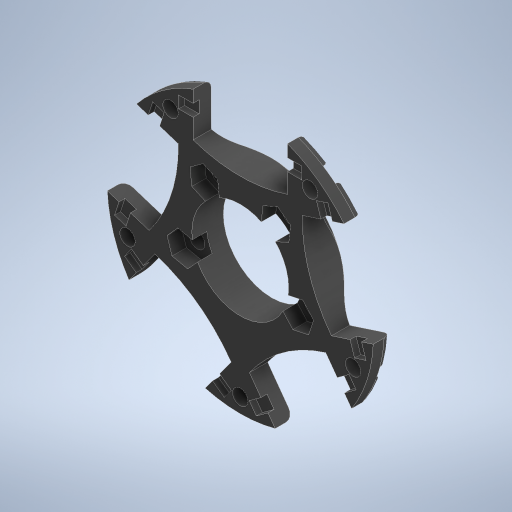
# Autodesk Inventor part: wheel_body_back_inside
Saved by Autodesk Inventor 2024.1 (Build 281209000, 209)
## iProperties
Created: 2024-11-26
Part Number: wheel_body_back_inside
Material: 一般
Document SubType Name: Modeling
Designer: hibik
Density: 1 g/cm^3
Appearance: 既定
Author: hibik
Autodesk Inventor part; units mm, degrees
ref_plane "YZ Plane" through (0, 0, 0) normal (1, 0, 0) x (0, 1, 0)
ref_plane "XZ Plane" through (0, 0, 0) normal (0, 1, 0) x (-1, 0, 0)
ref_plane "XY Plane" through (0, 0, 0) normal (0, 0, 1) x (1, 0, 0)
sketch "スケッチ1" plane through (0, 0, 0) normal (0, 0, 1) x (1, 0, 0)
  arc A0 (-9.75, 17.688144) -> (9.75, 17.688144) centre (0, 45) ccw
  arc A1 (-9.75, 16.62858) -> (9.75, 16.62858) centre (0, 45) ccw
  line L0 (-9.75, 42) -> (9.75, 42)
  line L1 (9.75, 42) -> (9.75, 15)
  line L2 (9.75, 15) -> (-9.75, 15)
  line L3 (-9.75, 15) -> (-9.75, 42)
  line L4 (-9.75, 29) -> (9.75, 29)
  circle A2 centre (0, 0) radius 10
  circle A3 centre (0, 0) radius 15 construction
  circle A4 centre (0, 0) radius 29
  line L5 (-17.278763, -4.637546) -> (-42.957289, 3.705913)
  arc A5 (-18.827635, -4.134287) -> (-12.801803, 14.411315) centre (-42.797543, 13.905765) ccw
  line L6 (-36.931458, 22.251515) -> (-11.252932, 13.908056)
  line L7 (-0.928863, -17.866161) -> (-16.799065, -39.70962)
  arc A6 (-1.886118, -19.18371) -> (-17.66195, -7.721897) centre (-26.450336, -36.405765) ccw
  line L8 (-32.574896, -28.247808) -> (-16.704694, -6.404349)
  line L9 (16.704694, -6.404349) -> (32.574896, -28.247808)
  arc A7 (17.66195, -7.721897) -> (1.886118, -19.18371) centre (26.450336, -36.405765) ccw
  line L10 (16.799065, -39.70962) -> (0.928863, -17.866161)
  line L11 (11.252932, 13.908056) -> (36.931458, 22.251515)
  arc A8 (12.801803, 14.411315) -> (18.827635, -4.134287) centre (42.797543, 13.905765) ccw
  line L12 (42.957289, 3.705913) -> (17.278763, -4.637546)
  circle A9 centre (0, 0) radius 27.5
  line L13 (-9.75, 16.62858) -> (-9.75, 27.311856)
  point P0 (0, 42)
  point P1 (-19.83534, -3.806864)
  point P2 (-24.567723, 18.234294)
  point P3 (-13.809509, 14.738738)
  point P4 (-2.508914, -20.040915)
  point P5 (-24.933688, -17.730587)
  point P6 (-18.284746, -8.579103)
  point P7 (18.284746, -8.579103)
  point P8 (9.157857, -29.192399)
  point P9 (2.508914, -20.040915)
  point P10 (13.809509, 14.738738)
  point P11 (30.593555, -0.311308)
  point P12 (19.83534, -3.806864)
  point P13 (9.75, 25.713566)
  point P14 (-9.75, 25.713566)
  point P15 (-21.442139, 17.21873)
  point P16 (-27.467971, -1.326872)
  point P17 (-23.001971, -15.071806)
  point P18 (-7.226139, -26.533618)
  point P19 (7.226139, -26.533618)
  point P20 (23.001971, -15.071806)
  point P21 (27.467971, -1.326872)
  point P22 (21.442139, 17.21873)
  point P23 (0, 15)
  point P24 (-9.75, 21.970218)
  dimension "d110" = 58
  dimension "d2" = 14
  dimension "d3" = 13
  dimension "d4" = 19.5
  dimension "d9" = 29
  dimension "d10" = 1
  dimension "d16" = 360
  dimension "d18" = 1.5
  dimension "d108" = 14
  dimension "d118" = 20
  constraints: 28 end point, 26 point on line, 12 point on circle, 9 centre point, 6 coincident, 2 horizontal, 2 midpoint, 2 parallel, 2 perpendicular, 2 tangent, 2 vertical alignment, 69 other
  measures "d2" distance between parallel lines of L2 L4
  measures "d3" distance between parallel lines of L0 L4
  measures "d4" distance of L0.start L0.end
  measures "d9" radius of A0
  measures "d10" radial gap between concentric circles of A0 A1
  measures "d118" diameter of A2
extrude "押し出し1" add sketch "スケッチ1" along normal blind 2.25 contours L3 L2 L1 A9 L11 A8 L12 L9 A7 L10 L7 A6 L8 L5 A5 L6 | A1 L2 L3 | L1 L2 A1
sketch "スケッチ2" plane through (0, 0, 2.25) normal (0, 0, 1) x (1, 0, 0)
  line L0 (-13.44258, 18.502125) -> (0, 0) construction
  line L1 (-9.75, 16.62858) -> (-9.75, 25.713566)
  line L2 (-21.442139, 17.21873) -> (-12.801803, 14.411315)
  arc A0 (-9.75, 25.713566) -> (-21.442139, 17.21873) centre (0, 0) ccw
  circle A1 centre (-14.400739, 19.820916) radius 1.6
  line L3 (-14.400739, 19.820916) -> (-16.744419, 18.118133)
  circle A2 centre (0, 0) radius 10
  circle A3 centre (0, 0) radius 24.5 construction
  circle A4 centre (-23.300885, -7.570916) radius 1.6
  circle A5 centre (0, -24.5) radius 1.6
  circle A6 centre (23.300885, -7.570916) radius 1.6
  circle A7 centre (14.400739, 19.820916) radius 1.6
  circle A8 centre (-7.347316, 10.112712) radius 1.6
  circle A9 centre (0, 0) radius 12.5 construction
  circle A10 centre (-11.888206, 3.862712) radius 1.6
  circle A11 centre (-11.888206, -3.862712) radius 1.6
  circle A12 centre (-7.347316, -10.112712) radius 1.6
  circle A13 centre (0, -12.5) radius 1.6
  circle A14 centre (7.347316, -10.112712) radius 1.6
  circle A15 centre (11.888206, -3.862712) radius 1.6
  circle A16 centre (11.888206, 3.862712) radius 1.6
  circle A17 centre (7.347316, 10.112712) radius 1.6
  circle A18 centre (0, 12.5) radius 1.6
  point P0 (-9.75, 57.7)
  point P1 (9.75, 25.713566)
  point P2 (-9.75, 17.688144)
  dimension "d123" = 25
  dimension "d22" = 36
  dimension "d23" = 36
  dimension "d34" = 20
  dimension "d111" = 3.2
  dimension "d113" = 3
  dimension "d116" = 360
  dimension "d122" = 3.2
  dimension "d126" = 360
  constraints: 15 centre point, 4 end point, 2 coincident, 2 point on line, 1 line through centre, 1 perpendicular, 38 other
  measures "d22" angle of L1 L0
  measures "d23" angle of L2 L0
  measures "d34" diameter of A2
  measures "d111" diameter of A1
  measures "d122" diameter of A8
extrude "押し出し2" cut sketch "スケッチ2" against normal through all contours A1 | A2 | A4 | A5 | A6 | A7 | A8 | A11 | A15 | A17
sketch "スケッチ3" plane through (0, 0, 2.25) normal (0, 0, 1) x (1, 0, 0)
  line L0 (-9.75, 20.680287) -> (-12.75, 20.680287)
  line L1 (-12.75, 20.680287) -> (-12.75, 23.180287)
  line L2 (-12.75, 23.180287) -> (-9.75, 23.180287)
  line L3 (-9.75, 23.180287) -> (-9.75, 20.680287)
  line L4 (9.75, 20.680287) -> (12.75, 20.680287)
  line L5 (12.75, 20.680287) -> (12.75, 23.180287)
  line L6 (12.75, 23.180287) -> (9.75, 23.180287)
  line L7 (9.75, 23.180287) -> (9.75, 20.680287)
  line L8 (-22.681038, -2.882241) -> (-23.608089, -5.73541)
  line L9 (-23.608089, -5.73541) -> (-25.98573, -4.962868)
  line L10 (-25.98573, -4.962868) -> (-25.058679, -2.109698)
  line L11 (-25.058679, -2.109698) -> (-22.681038, -2.882241)
  line L12 (-19.032848, 16.435904) -> (-16.655206, 15.663361)
  line L13 (-16.655206, 15.663361) -> (-15.728155, 18.516531)
  line L14 (-15.728155, 18.516531) -> (-18.105797, 19.289073)
  line L15 (-18.105797, 19.289073) -> (-19.032848, 16.435904)
  line L16 (-4.267652, -22.46161) -> (-1.840601, -24.224966)
  line L17 (-1.840601, -24.224966) -> (-3.310064, -26.247508)
  line L18 (-3.310064, -26.247508) -> (-5.737115, -24.484153)
  line L19 (-5.737115, -24.484153) -> (-4.267652, -22.46161)
  line L20 (-21.512947, -13.02234) -> (-20.043484, -10.999798)
  line L21 (-20.043484, -10.999798) -> (-22.470535, -9.236442)
  line L22 (-22.470535, -9.236442) -> (-23.939998, -11.258984)
  line L23 (-23.939998, -11.258984) -> (-21.512947, -13.02234)
  line L24 (20.043484, -10.999798) -> (22.470535, -9.236442)
  line L25 (22.470535, -9.236442) -> (23.939998, -11.258984)
  line L26 (23.939998, -11.258984) -> (21.512947, -13.02234)
  line L27 (21.512947, -13.02234) -> (20.043484, -10.999798)
  line L28 (5.737115, -24.484153) -> (4.267652, -22.46161)
  line L29 (4.267652, -22.46161) -> (1.840601, -24.224966)
  line L30 (1.840601, -24.224966) -> (3.310064, -26.247508)
  line L31 (3.310064, -26.247508) -> (5.737115, -24.484153)
  line L32 (16.655206, 15.663361) -> (15.728155, 18.516531)
  line L33 (15.728155, 18.516531) -> (18.105797, 19.289073)
  line L34 (18.105797, 19.289073) -> (19.032848, 16.435904)
  line L35 (19.032848, 16.435904) -> (16.655206, 15.663361)
  line L36 (25.058679, -2.109698) -> (22.681038, -2.882241)
  line L37 (22.681038, -2.882241) -> (23.608089, -5.73541)
  line L38 (23.608089, -5.73541) -> (25.98573, -4.962868)
  line L39 (25.98573, -4.962868) -> (25.058679, -2.109698)
  line L40 (-9.75, 16.62858) -> (-9.75, 25.713566)
  line L41 (9.75, 25.713566) -> (9.75, 16.62858)
  arc A0 (-12.800739, 19.820916) -> (-12.800739, 19.820916) centre (-14.400739, 19.820916) ccw
  circle A1 centre (0, 0) radius 24
  circle A2 centre (0, 0) radius 10
  point P0 (-9.75, 21.930287)
  point P1 (-23.869858, -2.49597)
  point P2 (-5.002384, -23.472881)
  point P3 (20.778215, -12.011069)
  point P4 (17.844027, 16.049632)
  point P5 (-9.75, 17.688144)
  point P6 (9.75, 17.688144)
  point P7 (9.75, 21.930287)
  dimension "d40" = 2.5
  dimension "d45" = 360
  dimension "d105" = 3
  dimension "d107" = 14
  constraints: 80 end point, 10 point on line, 4 parallel, 3 collinear, 2 horizontal, 2 midpoint, 2 perpendicular, 1 coincident, 1 horizontal alignment, 89 other
  measures "d40" distance of L0.end L1.end
  measures "d105" distance of L1.end L2.end
extrude "押し出し3" cut sketch "スケッチ3" against normal blind 1.25 contours L0 A1 L3 | L0 L1 L2 L3 A1 | A1 L4 L7 | L7 L6 L5 L4 A1 | A1 L12 L15 L14 L13 | L13 L12 A1 | A1 L35 L32 | L32 L33 L34 L35 A1 | A1 L8 L9 L10 L11 | L11 L8 A1 | A1 L37 L36 | L36 L39 L38 L37 A1 | A1 L20 L23 L22 L21 | L21 L20 A1 | A1 L27 L24 | L24 L25 L26 L27 A1 | A1 L16 L17 L18 L19 | L19 L16 A1 | A1 L29 L28 | L28 L31 L30 L29 A1
sketch "スケッチ13" plane through (0, 0, 0) normal (0, 0, -1) x (-1, 0, 0)
  circle A0 centre (14.400739, 19.820916) radius 1.6
  circle A1 centre (0, 0) radius 10
  circle A2 centre (0, 0) radius 16.5
  circle A3 centre (0, 0) radius 10
  circle A4 centre (14.400739, 19.820916) radius 1.6
  line L0 (-9.75, 23.180287) -> (-12.75, 23.180287)
  line L1 (-12.75, 23.180287) -> (-12.75, 20.680287)
  line L2 (-12.75, 20.680287) -> (-9.75, 20.680287)
  line L3 (9.75, 20.680287) -> (12.75, 20.680287)
  line L4 (12.75, 20.680287) -> (12.75, 23.180287)
  line L5 (12.75, 23.180287) -> (9.75, 23.180287)
  line L6 (4.267652, -22.46161) -> (1.840601, -24.224966)
  line L7 (1.840601, -24.224966) -> (3.310064, -26.247508)
  line L8 (3.310064, -26.247508) -> (5.737115, -24.484153)
  line L9 (-5.737115, -24.484153) -> (-3.310064, -26.247508)
  line L10 (-3.310064, -26.247508) -> (-1.840601, -24.224966)
  line L11 (-1.840601, -24.224966) -> (-4.267652, -22.46161)
  line L12 (9.75, 16.62858) -> (9.75, 25.713566)
  line L13 (-9.75, 25.713566) -> (-9.75, 16.62858)
  arc A5 (-9.75, 25.713566) -> (-21.442139, 17.21873) centre (0, 0) ccw
  line L14 (-12.801803, 14.411315) -> (-21.442139, 17.21873)
  arc A6 (-18.827635, -4.134287) -> (-12.801803, 14.411315) centre (-42.797543, 13.905765) ccw
  line L15 (-27.467971, -1.326872) -> (-18.827635, -4.134287)
  arc A7 (-27.467971, -1.326872) -> (-23.001971, -15.071806) centre (0, 0) ccw
  line L16 (-17.66195, -7.721897) -> (-23.001971, -15.071806)
  arc A8 (-1.886118, -19.18371) -> (-17.66195, -7.721897) centre (-26.450336, -36.405765) ccw
  line L17 (-7.226139, -26.533618) -> (-1.886118, -19.18371)
  arc A9 (-7.226139, -26.533618) -> (7.226139, -26.533618) centre (0, 0) ccw
  line L18 (1.886118, -19.18371) -> (7.226139, -26.533618)
  arc A10 (17.66195, -7.721897) -> (1.886118, -19.18371) centre (26.450336, -36.405765) ccw
  line L19 (23.001971, -15.071806) -> (17.66195, -7.721897)
  arc A11 (23.001971, -15.071806) -> (27.467971, -1.326872) centre (0, 0) ccw
  line L20 (18.827635, -4.134287) -> (27.467971, -1.326872)
  arc A12 (12.801803, 14.411315) -> (18.827635, -4.134287) centre (42.797543, 13.905765) ccw
  line L21 (21.442139, 17.21873) -> (12.801803, 14.411315)
  line L22 (-4.267652, -22.46161) -> (-1.886118, -19.18371)
  arc A13 (-1.886118, -19.18371) -> (-17.66195, -7.721897) centre (-26.450336, -36.405765) ccw
  line L23 (-17.66195, -7.721897) -> (-20.043484, -10.999798)
  line L24 (-20.043484, -10.999798) -> (-22.470535, -9.236442)
  line L25 (-22.470535, -9.236442) -> (-23.939998, -11.258984)
  line L26 (-23.939998, -11.258984) -> (-21.512947, -13.02234)
  line L27 (-21.512947, -13.02234) -> (-23.001971, -15.071806)
  arc A14 (-27.467971, -1.326872) -> (-23.001971, -15.071806) centre (0, 0) ccw
  line L28 (-27.467971, -1.326872) -> (-25.058679, -2.109698)
  line L29 (-25.058679, -2.109698) -> (-25.98573, -4.962868)
  line L30 (-25.98573, -4.962868) -> (-23.608089, -5.73541)
  line L31 (-23.608089, -5.73541) -> (-22.681038, -2.882241)
  line L32 (-22.681038, -2.882241) -> (-18.827635, -4.134287)
  arc A15 (-18.827635, -4.134287) -> (-12.801803, 14.411315) centre (-42.797543, 13.905765) ccw
  line L33 (-12.801803, 14.411315) -> (-16.655206, 15.663361)
  line L34 (-16.655206, 15.663361) -> (-15.728155, 18.516531)
  line L35 (-15.728155, 18.516531) -> (-18.105797, 19.289073)
  line L36 (-18.105797, 19.289073) -> (-19.032848, 16.435904)
  line L37 (-19.032848, 16.435904) -> (-21.442139, 17.21873)
  line L38 (-9.75, 25.713566) -> (-9.75, 23.180287)
  line L39 (-9.75, 20.680287) -> (-9.75, 16.62858)
  line L40 (9.75, 16.62858) -> (9.75, 20.680287)
  line L41 (9.75, 23.180287) -> (9.75, 25.713566)
  arc A16 (21.442139, 17.21873) -> (9.75, 25.713566) centre (0, 0) ccw
  line L42 (21.442139, 17.21873) -> (19.032848, 16.435904)
  line L43 (19.032848, 16.435904) -> (18.105797, 19.289073)
  line L44 (18.105797, 19.289073) -> (15.728155, 18.516531)
  line L45 (15.728155, 18.516531) -> (16.655206, 15.663361)
  line L46 (16.655206, 15.663361) -> (12.801803, 14.411315)
  arc A17 (12.801803, 14.411315) -> (18.827635, -4.134287) centre (42.797543, 13.905765) ccw
  line L47 (18.827635, -4.134287) -> (22.681038, -2.882241)
  line L48 (22.681038, -2.882241) -> (23.608089, -5.73541)
  line L49 (23.608089, -5.73541) -> (25.98573, -4.962868)
  line L50 (25.98573, -4.962868) -> (25.058679, -2.109698)
  line L51 (25.058679, -2.109698) -> (27.467971, -1.326872)
  arc A18 (23.001971, -15.071806) -> (27.467971, -1.326872) centre (0, 0) ccw
  line L52 (23.001971, -15.071806) -> (21.512947, -13.02234)
  line L53 (21.512947, -13.02234) -> (23.939998, -11.258984)
  line L54 (23.939998, -11.258984) -> (22.470535, -9.236442)
  line L55 (22.470535, -9.236442) -> (20.043484, -10.999798)
  line L56 (20.043484, -10.999798) -> (17.66195, -7.721897)
  arc A19 (17.66195, -7.721897) -> (1.886118, -19.18371) centre (26.450336, -36.405765) ccw
  line L57 (1.886118, -19.18371) -> (4.267652, -22.46161)
  line L58 (5.737115, -24.484153) -> (7.226139, -26.533618)
  arc A20 (-7.226139, -26.533618) -> (7.226139, -26.533618) centre (0, 0) ccw
  line L59 (-7.226139, -26.533618) -> (-5.737115, -24.484153)
  arc A21 (21.442139, 17.21873) -> (9.75, 25.713566) centre (0, 0) ccw
  arc A22 (-9.75, 25.713566) -> (-21.442139, 17.21873) centre (0, 0) ccw
  arc A23 (-9.75, 16.62858) -> (9.75, 16.62858) centre (0, 45) ccw
  arc A24 (-9.75, 16.62858) -> (9.75, 16.62858) centre (0, 45) ccw
  circle A25 centre (7.347316, 10.112712) radius 1.6
  circle A26 centre (0, 12.5) radius 1.6
  circle A27 centre (-7.347316, 10.112712) radius 1.6
  circle A28 centre (-11.888206, 3.862712) radius 1.6
  circle A29 centre (-11.888206, -3.862712) radius 1.6
  circle A30 centre (-7.347316, -10.112712) radius 1.6
  circle A31 centre (0, -12.5) radius 1.6
  circle A32 centre (7.347316, -10.112712) radius 1.6
  circle A33 centre (11.888206, -3.862712) radius 1.6
  circle A34 centre (11.888206, 3.862712) radius 1.6
  circle A35 centre (0, 0) radius 15
  arc A36 (12.801803, 14.411315) -> (18.827635, -4.134287) centre (42.797543, 13.905765) ccw
  point P0 (13.038403, 10.111876)
  point P1 (16.491902, -0.516898)
  point P2 (-13.038403, 10.111876)
  point P3 (-16.491902, -0.516898)
  point P4 (-13.646054, -9.275517)
  point P5 (-4.604678, -15.844461)
  point P6 (4.604678, -15.844461)
  point P7 (13.646054, -9.275517)
  point P8 (12.801803, 14.411315)
  point P9 (-12.801803, 14.411315)
  point P10 (-18.827635, -4.134287)
  point P11 (-17.66195, -7.721897)
  point P12 (-1.886118, -19.18371)
  point P13 (1.886118, -19.18371)
  point P14 (17.66195, -7.721897)
  point P15 (18.827635, -4.134287)
  point P16 (5.587878, 15.525)
  point P17 (-5.587878, 15.525)
  dimension "d136" = 1.5
  constraints: 2 centre point, 2 coincident, 1 tangent
  measures "d136" radial gap between concentric circles of A2 A35
extrude "押し出し13" add sketch "スケッチ13" along normal blind 4.25 contours A35 | A12 A2 A10 A35 | A12 A35 A23 A2 | A23 A35 A6 A2 | A2 A8 A35 A10 | A35 A8 A2 A6 | A26 | A28 | A30 | A31 | A32 | A34
sketch "スケッチ15" plane through (0, 0, 2.25) normal (0, 0, 1) x (1, 0, 0)
  circle A0 centre (-11.888206, -3.862712) radius 1.6
  circle A1 centre (-7.347316, 10.112712) radius 1.6
  circle A2 centre (7.347316, 10.112712) radius 1.6
  circle A3 centre (11.888206, -3.862712) radius 1.6
  circle A4 centre (0, -12.5) radius 1.6
  line L0 (1.659882, -9.625) -> (3.319764, -12.5)
  line L1 (3.319764, -12.5) -> (1.659882, -15.375)
  line L2 (1.659882, -15.375) -> (-1.659882, -15.375)
  line L3 (-1.659882, -15.375) -> (-3.319764, -12.5)
  line L4 (-3.319764, -12.5) -> (-1.659882, -9.625)
  line L5 (-1.659882, -9.625) -> (1.659882, -9.625)
  line L6 (0, 36.35628) -> (0, -38.142713)
  line L7 (-38.455159, 0) -> (38.455159, 0)
  line L8 (9.666851, -1.395647) -> (12.91407, -0.705429)
  line L9 (12.91407, -0.705429) -> (15.135426, -3.172495)
  line L10 (15.135426, -3.172495) -> (14.109562, -6.329778)
  line L11 (14.109562, -6.329778) -> (10.862343, -7.019996)
  line L12 (10.862343, -7.019996) -> (8.640987, -4.55293)
  line L13 (8.640987, -4.55293) -> (9.666851, -1.395647)
  line L14 (4.31456, 8.762443) -> (4.66157, 12.064021)
  line L15 (4.66157, 12.064021) -> (7.694325, 13.41429)
  line L16 (7.694325, 13.41429) -> (10.380071, 11.462982)
  line L17 (10.380071, 11.462982) -> (10.033061, 8.161404)
  line L18 (10.033061, 8.161404) -> (7.000306, 6.811134)
  line L19 (7.000306, 6.811134) -> (4.31456, 8.762443)
  line L20 (-7.000306, 6.811134) -> (-10.033061, 8.161404)
  line L21 (-10.033061, 8.161404) -> (-10.380071, 11.462982)
  line L22 (-10.380071, 11.462982) -> (-7.694325, 13.41429)
  line L23 (-7.694325, 13.41429) -> (-4.66157, 12.064021)
  line L24 (-4.66157, 12.064021) -> (-4.31456, 8.762443)
  line L25 (-4.31456, 8.762443) -> (-7.000306, 6.811134)
  line L26 (-8.640987, -4.55293) -> (-10.862343, -7.019996)
  line L27 (-10.862343, -7.019996) -> (-14.109562, -6.329778)
  line L28 (-14.109562, -6.329778) -> (-15.135426, -3.172495)
  line L29 (-15.135426, -3.172495) -> (-12.91407, -0.705429)
  line L30 (-12.91407, -0.705429) -> (-9.666851, -1.395647)
  line L31 (-9.666851, -1.395647) -> (-8.640987, -4.55293)
  point P0 (0, 0)
  point P1 (11.888206, -3.862712)
  point P2 (7.347316, 10.112712)
  point P3 (-7.347316, 10.112712)
  point P4 (-11.888206, -3.862712)
  dimension "d131" = 5.75
  dimension "d134" = 360
  constraints: 60 end point, 1 coincident, 1 midpoint, 1 perpendicular, 1 point on line, 79 other
  measures "d131" distance between parallel lines of L2 L5
extrude "押し出し15" cut sketch "スケッチ15" against normal blind 3 contours A0 | A1 | A2 | A3 | L8 L9 L10 L11 L12 L13 | L14 L15 L16 L17 L18 L19 | L20 L21 L22 L23 L24 L25 | L26 L27 L28 L29 L30 L31
chamfer "面取り1" distance 1.5 angle 45 5 edges at (15.6924, -5.0988, -4.25) (9.6985, 13.3488, -4.25) (-9.6985, 13.3488, -4.25) (-15.6924, -5.0988, -4.25) (0, -16.5, -4.25)
sketch "スケッチ16" plane through (0, 0, -4.25) normal (0, 0, -1) x (-1, 0, 0)
  circle A0 centre (0, 0) radius 12
  circle A1 centre (0, 10) radius 2
  line L0 (0, 0) -> (0, 10)
  circle A2 centre (-10, 0) radius 2
  circle A3 centre (0, -10) radius 2
  circle A4 centre (10, 0) radius 2
  circle A5 centre (0, 0) radius 3
  line L1 (-1.989975, -10.2) -> (-2.984962, -0.3)
  line L2 (2.984962, -0.3) -> (1.989975, -10.2)
  line L3 (0.3, 2.984962) -> (10.2, 1.989975)
  line L4 (10.2, -1.989975) -> (0.3, -2.984962)
  line L5 (-2.984962, 0.3) -> (-1.989975, 10.2)
  line L6 (1.989975, 10.2) -> (2.984962, 0.3)
  line L7 (-0.3, -2.984962) -> (-10.2, -1.989975)
  line L8 (-10.2, 1.989975) -> (-0.3, 2.984962)
  point P0 (2.739757, -2.739757)
  point P1 (2.739757, 2.739757)
  point P2 (-2.739757, 2.739757)
  point P3 (-2.739757, -2.739757)
  dimension "d141" = 24
  dimension "d142" = 4
  dimension "d145" = 360
  dimension "d147" = 6
  dimension "d150" = 360
  constraints: 18 end point, 6 centre point, 5 tangent, 4 point on circle, 3 coincident, 1 vertical alignment, 34 other
  measures "d141" diameter of A0
  measures "d142" diameter of A1
  measures "d147" diameter of A5
sketch "スケッチ17" plane through (0, 0, 0) normal (0, 0, -1) x (-1, 0, 0)
  circle A0 centre (0, -24.5) radius 1.6
  arc A1 (-4.604678, -15.844461) -> (4.604678, -15.844461) centre (0, 0) ccw
  arc A2 (-1.886118, -19.18371) -> (-4.604678, -15.844461) centre (-26.450336, -36.405765) ccw
  line L0 (-7.226139, -26.533618) -> (-1.886118, -19.18371)
  arc A3 (-7.226139, -26.533618) -> (7.226139, -26.533618) centre (0, 0) ccw
  line L1 (1.886118, -19.18371) -> (7.226139, -26.533618)
  arc A4 (4.604678, -15.844461) -> (1.886118, -19.18371) centre (26.450336, -36.405765) ccw
  line L2 (-1.645448, -27.35) -> (-3.290897, -24.5)
  line L3 (-3.290897, -24.5) -> (-1.645448, -21.65)
  line L4 (-1.645448, -21.65) -> (1.645448, -21.65)
  line L5 (1.645448, -21.65) -> (3.290897, -24.5)
  line L6 (3.290897, -24.5) -> (1.645448, -27.35)
  line L7 (1.645448, -27.35) -> (-1.645448, -27.35) construction
  line L8 (-1.645448, -27.35) -> (-1.585247, -27.454271)
  line L9 (1.645448, -27.35) -> (1.585247, -27.454271)
  line L10 (20.081902, -8.255132) -> (21.098845, -5.125304)
  line L11 (21.098845, -5.125304) -> (24.317828, -4.441088)
  line L12 (22.283942, -10.700745) -> (20.081902, -8.255132)
  line L13 (24.317828, -4.441088) -> (26.519867, -6.8867)
  line L14 (26.519867, -6.8867) -> (26.600432, -6.976176)
  line L15 (26.519867, -6.8867) -> (25.502924, -10.016529) construction
  line L16 (25.502924, -10.016529) -> (25.620695, -9.991496)
  line L17 (25.502924, -10.016529) -> (22.283942, -10.700745)
  line L18 (14.056746, 16.548048) -> (11.394355, 18.482388)
  line L19 (11.394355, 18.482388) -> (11.738347, 21.755257)
  line L20 (17.06313, 17.886576) -> (14.056746, 16.548048)
  line L21 (11.738347, 21.755257) -> (14.744731, 23.093785)
  line L22 (14.744731, 23.093785) -> (14.854723, 23.142757)
  line L23 (14.744731, 23.093785) -> (17.407122, 21.159445) construction
  line L24 (17.407122, 21.159445) -> (17.419708, 21.279187)
  line L25 (17.407122, 21.159445) -> (17.06313, 17.886576)
  line L26 (-11.394355, 18.482388) -> (-14.056746, 16.548048)
  line L27 (-14.056746, 16.548048) -> (-17.06313, 17.886576)
  line L28 (-11.738347, 21.755257) -> (-11.394355, 18.482388)
  line L29 (-17.06313, 17.886576) -> (-17.407122, 21.159445)
  line L30 (-17.407122, 21.159445) -> (-17.419708, 21.279187)
  line L31 (-17.407122, 21.159445) -> (-14.744731, 23.093785) construction
  line L32 (-14.744731, 23.093785) -> (-14.854723, 23.142757)
  line L33 (-14.744731, 23.093785) -> (-11.738347, 21.755257)
  line L34 (-21.098845, -5.125304) -> (-20.081902, -8.255132)
  line L35 (-20.081902, -8.255132) -> (-22.283942, -10.700745)
  line L36 (-24.317828, -4.441088) -> (-21.098845, -5.125304)
  line L37 (-22.283942, -10.700745) -> (-25.502924, -10.016529)
  line L38 (-25.502924, -10.016529) -> (-25.620695, -9.991496)
  line L39 (-25.502924, -10.016529) -> (-26.519867, -6.8867) construction
  line L40 (-26.519867, -6.8867) -> (-26.600432, -6.976176)
  line L41 (-26.519867, -6.8867) -> (-24.317828, -4.441088)
  circle A5 centre (23.300885, -7.570916) radius 1.6
  arc A6 (13.646054, -9.275517) -> (16.491902, -0.516898) centre (0, 0) ccw
  arc A7 (17.66195, -7.721897) -> (13.646054, -9.275517) centre (26.450336, -36.405765) ccw
  line L42 (23.001971, -15.071806) -> (17.66195, -7.721897)
  arc A8 (23.001971, -15.071806) -> (27.467971, -1.326872) centre (0, 0) ccw
  line L43 (18.827635, -4.134287) -> (27.467971, -1.326872)
  arc A9 (16.491902, -0.516898) -> (18.827635, -4.134287) centre (42.797543, 13.905765) ccw
  arc A10 (13.038403, 10.111876) -> (5.587878, 15.525) centre (0, 0) ccw
  arc A11 (12.801803, 14.411315) -> (13.038403, 10.111876) centre (42.797543, 13.905765) ccw
  line L44 (21.442139, 17.21873) -> (12.801803, 14.411315)
  arc A12 (21.442139, 17.21873) -> (9.75, 25.713566) centre (0, 0) ccw
  line L45 (9.75, 16.62858) -> (9.75, 25.713566)
  arc A13 (5.587878, 15.525) -> (9.75, 16.62858) centre (0, 45) ccw
  circle A14 centre (14.400739, 19.820916) radius 1.6
  circle A15 centre (-14.400739, 19.820916) radius 1.6
  arc A16 (-5.587878, 15.525) -> (-13.038403, 10.111876) centre (0, 0) ccw
  arc A17 (-9.75, 16.62858) -> (-5.587878, 15.525) centre (0, 45) ccw
  line L46 (-9.75, 25.713566) -> (-9.75, 16.62858)
  arc A18 (-9.75, 25.713566) -> (-21.442139, 17.21873) centre (0, 0) ccw
  line L47 (-12.801803, 14.411315) -> (-21.442139, 17.21873)
  arc A19 (-13.038403, 10.111876) -> (-12.801803, 14.411315) centre (-42.797543, 13.905765) ccw
  circle A20 centre (-23.300885, -7.570916) radius 1.6
  arc A21 (-16.491902, -0.516898) -> (-13.646054, -9.275517) centre (0, 0) ccw
  arc A22 (-18.827635, -4.134287) -> (-16.491902, -0.516898) centre (-42.797543, 13.905765) ccw
  line L48 (-27.467971, -1.326872) -> (-18.827635, -4.134287)
  arc A23 (-27.467971, -1.326872) -> (-23.001971, -15.071806) centre (0, 0) ccw
  line L49 (-17.66195, -7.721897) -> (-23.001971, -15.071806)
  arc A24 (-13.646054, -9.275517) -> (-17.66195, -7.721897) centre (-26.450336, -36.405765) ccw
  point P0 (16.491902, -0.516898)
  point P1 (13.646054, -9.275517)
  point P2 (18.827635, -4.134287)
  point P3 (23.300885, -7.570916)
  point P4 (23.300885, -7.570916)
  point P5 (27.467971, -1.326872)
  point P6 (23.001971, -15.071806)
  point P7 (17.66195, -7.721897)
  point P8 (5.587878, 15.525)
  point P9 (13.038403, 10.111876)
  point P10 (9.75, 16.62858)
  point P11 (14.400739, 19.820916)
  point P12 (14.400739, 19.820916)
  point P13 (9.75, 25.713566)
  point P14 (21.442139, 17.21873)
  point P15 (12.801803, 14.411315)
  point P16 (-13.038403, 10.111876)
  point P17 (-5.587878, 15.525)
  point P18 (-12.801803, 14.411315)
  point P19 (-14.400739, 19.820916)
  point P20 (-14.400739, 19.820916)
  point P21 (-21.442139, 17.21873)
  point P22 (-9.75, 25.713566)
  point P23 (-9.75, 16.62858)
  point P24 (-13.646054, -9.275517)
  point P25 (-16.491902, -0.516898)
  point P26 (-17.66195, -7.721897)
  point P27 (-23.300885, -7.570916)
  point P28 (-23.300885, -7.570916)
  point P29 (-23.001971, -15.071806)
  point P30 (-27.467971, -1.326872)
  point P31 (-18.827635, -4.134287)
  dimension "d154" = 5.7
  dimension "d157" = 360
  constraints: 80 end point, 5 coincident, 2 collinear, 2 point on circle, 1 horizontal, 134 other
  measures "d154" distance between parallel lines of L7 L4
extrude "押し出し17" add sketch "スケッチ17" along normal blind 1.5 contours A1 A4 L1 A3 L9 L6 L5 L4 L3 L2 L8 L0 A2 | L12 L17 L16 A8 L42 A7 A6 A9 L43 L14 L13 L11 L10 | L20 L25 L24 A12 L44 A11 A10 A13 L45 L22 L21 L19 L18 | L28 L33 L32 A18 L46 A17 A16 A19 L47 L30 L29 L27 L26 | L36 L41 L40 A23 L48 A22 A21 A24 L49 L38 L37 L35 L34
fillet "フィレット10" radius 5 5 edges at (-9.6985, 13.3488, -1.5) (-15.6924, -5.0988, -1.5) (0, -16.5, -1.5) (15.6924, -5.0988, -1.5) (9.6985, 13.3488, -1.5)
fillet "フィレット11" radius 1.5 10 edges at (12.3693, 24.5611, -1.5) (19.5367, 19.3537, -1.5) (27.1814, -4.1741, -1.5) (24.4437, -12.5999, -1.5) (4.4297, -27.1409, -1.5) (-4.4297, -27.1409, -1.5) (-24.4437, -12.5999, -1.5) (-27.1814, -4.1741, -1.5) (-19.5367, 19.3537, -1.5) (-12.3693, 24.5611, -1.5)
equation "\"d22\" = d23"
